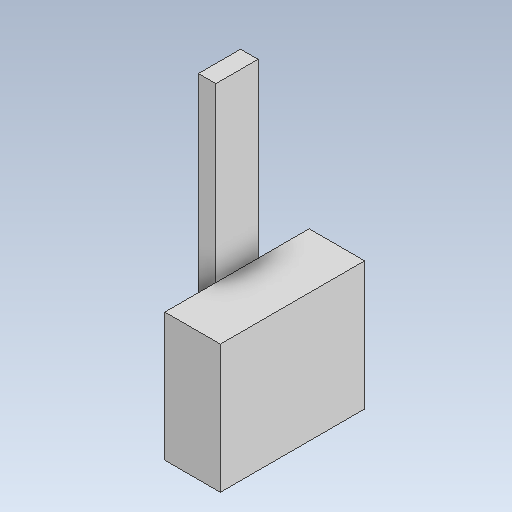
# Autodesk Inventor part: Test1
Saved by Autodesk Inventor 2025.2 (Build 292293000, 293)
## iProperties
Created: 2025-05-19
Part Number: Test1
Material: Generic
Document SubType Name: Modeling
Designer: Sergio Quintero
Mass: 48107.3 g
Surface Area: 8741.01 cm^2
Volume: 48107.3 cm^3
Density: 1 g/cm^3
Appearance: Default
Author: Sergio Quintero
Autodesk Inventor part; units mm, degrees
ref_plane "YZ Plane" through (0, 0, 0) normal (1, 0, 0) x (0, 1, 0)
ref_plane "XZ Plane" through (0, 0, 0) normal (0, 1, 0) x (-1, 0, 0)
ref_plane "XY Plane" through (0, 0, 0) normal (0, 0, 1) x (1, 0, 0)
sketch "Sketch1" plane through (0, 0, 0) normal (0, 1, 0) x (-1, 0, 0)
  line L0 (-100, -260) -> (100, -260)
  line L1 (100, -260) -> (100, 260)
  line L2 (100, 260) -> (-100, 260)
  line L3 (-100, 260) -> (-100, -260)
  line L4 (-100, -260) -> (100, 260) construction
  line L5 (100, -260) -> (-100, 260) construction
  point P0 (0, 0)
  dimension "d0" = 200
  dimension "d1" = 520
  constraints: 12 end point, 2 midpoint, 2 parallel, 1 horizontal, 1 perpendicular
  measures "d0" distance of L2.end L1.end
  measures "d1" distance of L1.end L0.end
extrude "Extrusion1" add sketch "Sketch1" along normal blind 462.57
sketch "Sketch2" plane through (0, 462.57, 0) normal (0, 1, 0) x (1, 0, 0)
  line L0 (-100, 260) -> (-100, -260) projected
  line L1 (-100, 76) -> (-163, 76)
  line L2 (-163, 76) -> (-163, -76)
  line L3 (-163, -76) -> (-100, -76)
  line L4 (-100, -76) -> (-100, 76)
  line L5 (-215.6, 0) -> (152.6, 0) projected
  point P0 (0, 0)
  dimension "d4" = 63
  dimension "d5" = 152
  constraints: 8 end point, 2 parallel, 1 horizontal, 1 perpendicular, 1 point on line, 1 other
  measures "d4" distance of L3.end L2.end
  measures "d5" distance of L2.end L1.end
extrude "Extrusion2" add sketch "Sketch2" along normal blind 621.1 and the other way blind 129 separate body
body "Solid1"
body "Solid2"
